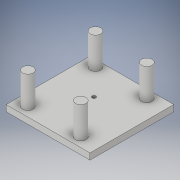
# Autodesk Inventor part: base1
Saved by Autodesk Inventor 2019 (Build 230136000, 136)
## iProperties
Created: 2020-02-20
Part Number: base1
Material: Generic
Document SubType Name: Modeling
Designer: ADMIN
Density: 1 g/cm^3
Appearance: Default
Author: ADMIN
Autodesk Inventor part; units mm, degrees
ref_plane "YZ Plane" through (0, 0, 0) normal (1, 0, 0) x (0, 1, 0)
ref_plane "XZ Plane" through (0, 0, 0) normal (0, 1, 0) x (-1, 0, 0)
ref_plane "XY Plane" through (0, 0, 0) normal (0, 0, 1) x (1, 0, 0)
sketch "Sketch1" plane through (0, 0, 0) normal (0, 1, 0) x (-1, 0, 0)
  line L0 (6.0199, 12.6049) -> (-393.9801, 12.6049)
  line L1 (-393.9801, 12.6049) -> (-393.9801, -387.3951)
  line L2 (-393.9801, -387.3951) -> (6.0199, -387.3951)
  line L3 (6.0199, -387.3951) -> (6.0199, 12.6049)
  point P0 (0, 0)
  dimension "d0" = 400
  dimension "d1" = 400
  dimension "d2" = 400
  constraints: 8 end point, 1 horizontal, 1 perpendicular, 1 vertical
  measures "d0" distance of L0.start L0.end
  measures "d1" distance of L0.end L1.end
  measures "d2" distance of L1.end L2.end
extrude "Extrusion1" add sketch "Sketch1" along normal blind 30
sketch "Sketch2" plane through (0, 30, 0) normal (0, 1, 0) x (1, 0, 0)
  circle A0 centre (52.6612, 32.1839) radius 25
  circle A1 centre (304.9932, 32.1839) radius 25
  circle A2 centre (304.9932, 347.5989) radius 25
  circle A3 centre (52.6612, 354.7675) radius 25
  point P0 (0, 0)
  dimension "d5" = 50
  dimension "d6" = 50
  dimension "d7" = 50
  dimension "d8" = 50
  constraints: 4 centre point
  measures "d5" diameter of A0
  measures "d6" diameter of A1
  measures "d7" diameter of A2
  measures "d8" diameter of A3
extrude "Extrusion2" add sketch "Sketch2" along normal blind 150
sketch "Sketch3" plane through (0, 0, 0) normal (0, -1, 0) x (1, 0, 0)
  point P0 (0, 0)
sketch "Sketch4" plane through (0, 30, 0) normal (0, 1, 0) x (1, 0, 0)
  point P0 (0, 0)
  point P1 (172.4185, 228.0493)
hole "Hole1" at (172.4185, 30, -228.0493) direction (0, -1, 0) diameter 17.894 depth 53.975 tip angle 118 thread size "13/16-10 UNC" class "2B" standard "ANSI Unified Screw Threads"
body "Solid1"
